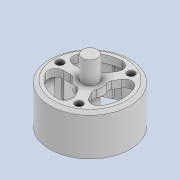
# Autodesk Inventor part: motor_1608_outer
Saved by Autodesk Inventor 2020 (Build 240168000, 168)
## iProperties
Created: 2020-01-30
Part Number: motor_1608_outer
Material: Generic
Document SubType Name: Modeling
Designer: psrobotics
Density: 1 g/cm^3
Appearance: Default
Author: psrobotics
Autodesk Inventor part; units mm, degrees
ref_plane "YZ Plane" through (0, 0, 0) normal (1, 0, 0) x (0, 1, 0)
ref_plane "XZ Plane" through (0, 0, 0) normal (0, 1, 0) x (-1, 0, 0)
ref_plane "XY Plane" through (0, 0, 0) normal (0, 0, 1) x (1, 0, 0)
sketch "Sketch1" plane through (0, 0, 0) normal (0, 1, 0) x (-1, 0, 0)
  circle A0 centre (0, 0) radius 8
  dimension "d0" = 16
  constraints: 1 centre point, 1 coincident
  measures "d0" diameter of A0
extrude "Extrusion1" add sketch "Sketch1" along normal blind 8
sketch "Sketch2" plane through (0, 8, 0) normal (0, 1, 0) x (1, 0, 0)
  circle A0 centre (0, 0) radius 8 projected
  circle A1 centre (0, 0) radius 1.5
  dimension "d3" = 3
  constraints: 1 centre point, 1 coincident
  measures "d3" diameter of A1
extrude "Extrusion2" add sketch "Sketch2" along normal blind 4.5 contours A1
sketch "Sketch3" plane through (0, 0, 0) normal (0, -1, 0) x (1, 0, 0)
  circle A0 centre (0, 0) radius 8 projected
  circle A1 centre (0, 0) radius 7.5
  dimension "d6" = 15
  constraints: 1 centre point, 1 coincident
  measures "d6" diameter of A1
extrude "Extrusion3" cut sketch "Sketch3" against normal blind 6.5 contours A1
sketch "Sketch4" plane through (0, 6.5, 0) normal (0, -1, 0) x (1, 0, 0)
  circle A0 centre (0, 0) radius 7.5 projected
  circle A1 centre (0, 0) radius 7
  line L0 (0, 0) -> (7.5, 0)
  circle A2 centre (0, 0) radius 7.5 projected
  line L1 (0, 0) -> (6.9038, -2.9305)
  point P0 (6.4435, -2.7351)
  point P1 (6.9038, -2.9305)
  point P2 (7, 0)
  dimension "d9" = 14
  dimension "d10" = 23
  constraints: 4 end point, 2 point on circle, 1 centre point, 1 coincident, 1 horizontal
  measures "d9" diameter of A1
  measures "d10" angle of L0 L1
extrude "Extrusion4" add sketch "Sketch4" along normal blind 6.2 contours A0 L1 A1 L0 picked at (6.8601, -2.5496)
pattern_circular "Circular Pattern1" count 10 over 360 about axis through (0, 0, 0) along (0, 1, 0) of "Extrusion4"
sketch "Sketch5" plane through (0, 8, 0) normal (0, 1, 0) x (1, 0, 0)
  circle A0 centre (0, 0) radius 2.5
  circle A1 centre (0, 0) radius 6.5
  line L0 (-10, -1) -> (-10, 1)
  line L1 (-10, 1) -> (10, 1)
  line L2 (10, 1) -> (10, -1)
  line L3 (10, -1) -> (-10, -1)
  line L4 (-10, -1) -> (10, 1) construction
  line L5 (-10, 1) -> (10, -1) construction
  line L6 (0, 0) -> (3.25, 5.6292)
  line L7 (0, 0) -> (-6.5, 0)
  line L8 (-5.866, -8.1603) -> (-4.134, -9.1603)
  line L9 (-4.134, -9.1603) -> (5.866, 8.1603)
  line L10 (5.866, 8.1603) -> (4.134, 9.1603)
  line L11 (4.134, 9.1603) -> (-5.866, -8.1603)
  line L12 (-5.866, -8.1603) -> (5.866, 8.1603) construction
  line L13 (-4.134, -9.1603) -> (4.134, 9.1603) construction
  point P0 (0.2796, 2.4843)
  point P1 (2.3453, 6.0621)
  point P2 (-6.4226, 1)
  point P3 (-2.2913, 1)
  dimension "d16" = 5
  dimension "d17" = 13
  dimension "d18" = 2
  dimension "d19" = 20
  dimension "d20" = 120
  dimension "d21" = 2
  dimension "d22" = 20
  constraints: 28 end point, 4 midpoint, 4 parallel, 3 perpendicular, 2 centre point, 2 coincident, 2 point on circle, 1 horizontal, 1 vertical
  measures "d16" diameter of A0
  measures "d17" diameter of A1
  measures "d18" distance of L0.start L0.end
  measures "d19" distance of L0.end L1.end
  measures "d20" angle of L7 L6
  measures "d21" distance of L8.start L8.end
  measures "d22" distance of L9.end L8.end
extrude "Extrusion5" cut sketch "Sketch5" against normal blind 6.2 contours A0 L1 A1 L11
pattern_circular "Circular Pattern2" count 3 over 360 about axis through (0, 8, 0) along (0, -1, 0) of "Extrusion5"
fillet "Fillet1" radius 1.5 2 edges at (-6.4226, 7.25, -1) (2.3453, 7.25, -6.0621)
pattern_circular "Circular Pattern3" count 3 over 360 about axis through (0, 8, 0) along (0, 1, 0) of "Fillet1"
fillet "Fillet2" radius 1 2 edges at (-2.2913, 7.25, -1) (0.2796, 7.25, -2.4843)
pattern_circular "Circular Pattern4" count 3 over 360 about axis through (0, 8, 0) along (0, 1, 0) of "Fillet2"
chamfer "Chamfer1" distance 0.8 angle 30 1 edges at (8, 8, 0) measured on face at (-6.1962, 8, 0)
sketch "Sketch6" plane through (0, 6.5, 0) normal (0, -1, 0) x (1, 0, 0)
  arc A0 (0, 6.5) -> (-5.6292, 3.25) centre (0, 0) ccw projected
  arc A1 (1.299, 4.25) -> (0, 6.5) centre (0, 5) ccw projected
  line L0 (1.299, 4.25) -> (0.5701, 2.9875) projected
  arc A2 (-0.2114, 2.491) -> (0.5701, 2.9875) centre (-0.2959, 3.4875) ccw projected
  arc A3 (-0.2114, 2.491) -> (-2.0516, 1.4286) centre (0, 0) ccw projected
  arc A4 (-2.8723, 1) -> (-2.0516, 1.4286) centre (-2.8723, 2) ccw projected
  line L1 (-2.8723, 1) -> (-4.3301, 1) projected
  arc A5 (-5.6292, 3.25) -> (-4.3301, 1) centre (-4.3301, 2.5) ccw projected
  arc A6 (5.6292, -3.25) -> (5.6292, 3.25) centre (0, 0) ccw projected
  arc A7 (3.0311, -3.25) -> (5.6292, -3.25) centre (4.3301, -2.5) ccw projected
  line L2 (3.0311, -3.25) -> (2.3022, -1.9875) projected
  arc A8 (2.263, -1.0625) -> (2.3022, -1.9875) centre (3.1682, -1.4875) ccw projected
  arc A9 (2.263, -1.0625) -> (2.263, 1.0625) centre (0, 0) ccw projected
  arc A10 (2.3022, 1.9875) -> (2.263, 1.0625) centre (3.1682, 1.4875) ccw projected
  line L3 (2.3022, 1.9875) -> (3.0311, 3.25) projected
  arc A11 (5.6292, 3.25) -> (3.0311, 3.25) centre (4.3301, 2.5) ccw projected
  arc A12 (-5.6292, -3.25) -> (0, -6.5) centre (0, 0) ccw projected
  arc A13 (-4.3301, -1) -> (-5.6292, -3.25) centre (-4.3301, -2.5) ccw projected
  line L4 (-4.3301, -1) -> (-2.8723, -1) projected
  arc A14 (-2.0516, -1.4286) -> (-2.8723, -1) centre (-2.8723, -2) ccw projected
  arc A15 (-2.0516, -1.4286) -> (-0.2114, -2.491) centre (0, 0) ccw projected
  arc A16 (0.5701, -2.9875) -> (-0.2114, -2.491) centre (-0.2959, -3.4875) ccw projected
  line L5 (0.5701, -2.9875) -> (1.299, -4.25) projected
  arc A17 (0, -6.5) -> (1.299, -4.25) centre (0, -5) ccw projected
  line L6 (7.3078, 1.6871) -> (6.8206, 1.5747) projected
  arc A18 (6.8206, 1.5747) -> (5.6631, 4.1145) centre (0, 0) ccw projected
  line L7 (5.6631, 4.1145) -> (6.0676, 4.4084) projected
  arc A19 (6.0676, 4.4084) -> (4.9204, 5.6603) centre (0, 0) ccw projected
  line L8 (4.9204, 5.6603) -> (4.5924, 5.283) projected
  arc A20 (4.5924, 5.283) -> (2.1631, 6.6574) centre (0, 0) ccw projected
  line L9 (2.1631, 6.6574) -> (2.3176, 7.1329) projected
  arc A21 (2.3176, 7.1329) -> (0.6537, 7.4715) centre (0, 0) ccw projected
  line L10 (0.6537, 7.4715) -> (0.6101, 6.9734) projected
  arc A22 (0.6101, 6.9734) -> (-2.1631, 6.6574) centre (0, 0) ccw projected
  line L11 (-2.1631, 6.6574) -> (-2.3176, 7.1329) projected
  arc A23 (-2.3176, 7.1329) -> (-3.8628, 6.4288) centre (0, 0) ccw projected
  line L12 (-3.8628, 6.4288) -> (-3.6053, 6.0002) projected
  arc A24 (-3.6053, 6.0002) -> (-5.6631, 4.1145) centre (0, 0) ccw projected
  line L13 (-5.6631, 4.1145) -> (-6.0676, 4.4084) projected
  arc A25 (-6.0676, 4.4084) -> (-6.9038, 2.9305) centre (0, 0) ccw projected
  line L14 (-6.9038, 2.9305) -> (-6.4435, 2.7351) projected
  arc A26 (-6.4435, 2.7351) -> (-7, 0) centre (0, 0) ccw projected
  line L15 (-7, 0) -> (-7.5, 0) projected
  arc A27 (-7.5, 0) -> (-7.3078, -1.6871) centre (0, 0) ccw projected
  line L16 (-7.3078, -1.6871) -> (-6.8206, -1.5747) projected
  arc A28 (-6.8206, -1.5747) -> (-5.6631, -4.1145) centre (0, 0) ccw projected
  line L17 (-5.6631, -4.1145) -> (-6.0676, -4.4084) projected
  arc A29 (-6.0676, -4.4084) -> (-4.9204, -5.6603) centre (0, 0) ccw projected
  line L18 (-4.9204, -5.6603) -> (-4.5924, -5.283) projected
  arc A30 (-4.5924, -5.283) -> (-2.1631, -6.6574) centre (0, 0) ccw projected
  line L19 (-2.1631, -6.6574) -> (-2.3176, -7.1329) projected
  arc A31 (-2.3176, -7.1329) -> (-0.6537, -7.4715) centre (0, 0) ccw projected
  line L20 (-0.6537, -7.4715) -> (-0.6101, -6.9734) projected
  arc A32 (-0.6101, -6.9734) -> (2.1631, -6.6574) centre (0, 0) ccw projected
  line L21 (2.1631, -6.6574) -> (2.3176, -7.1329) projected
  arc A33 (2.3176, -7.1329) -> (3.8628, -6.4288) centre (0, 0) ccw projected
  line L22 (3.8628, -6.4288) -> (3.6053, -6.0002) projected
  arc A34 (3.6053, -6.0002) -> (5.6631, -4.1145) centre (0, 0) ccw projected
  line L23 (5.6631, -4.1145) -> (6.0676, -4.4084) projected
  arc A35 (6.0676, -4.4084) -> (6.9038, -2.9305) centre (0, 0) ccw projected
  line L24 (6.9038, -2.9305) -> (6.4435, -2.7351) projected
  arc A36 (6.4435, -2.7351) -> (7, 0) centre (0, 0) ccw projected
  line L25 (7, 0) -> (7.5, 0) projected
  arc A37 (7.5, 0) -> (7.3078, 1.6871) centre (0, 0) ccw projected
  circle A38 centre (0, 0) radius 1.5
  dimension "d39" = 3
  constraints: 1 centre point, 1 coincident
  measures "d39" diameter of A38
extrude "Extrusion6" add sketch "Sketch6" along normal blind 5 contours A38
sketch "Sketch7" plane through (0, 8, 0) normal (0, 1, 0) x (1, 0, 0)
  circle A0 centre (0, 0) radius 1.5 projected
  arc A1 (0, 6.5) -> (-5.6292, 3.25) centre (0, 0) ccw projected
  arc A2 (1.299, 4.25) -> (0, 6.5) centre (0, 5) ccw projected
  line L0 (1.299, 4.25) -> (0.5701, 2.9875) projected
  arc A3 (-0.2114, 2.491) -> (0.5701, 2.9875) centre (-0.2959, 3.4875) ccw projected
  arc A4 (-0.2114, 2.491) -> (-2.0516, 1.4286) centre (0, 0) ccw projected
  arc A5 (-2.8723, 1) -> (-2.0516, 1.4286) centre (-2.8723, 2) ccw projected
  line L1 (-2.8723, 1) -> (-4.3301, 1) projected
  arc A6 (-5.6292, 3.25) -> (-4.3301, 1) centre (-4.3301, 2.5) ccw projected
  arc A7 (5.6292, -3.25) -> (5.6292, 3.25) centre (0, 0) ccw projected
  arc A8 (3.0311, -3.25) -> (5.6292, -3.25) centre (4.3301, -2.5) ccw projected
  line L2 (3.0311, -3.25) -> (2.3022, -1.9875) projected
  arc A9 (2.263, -1.0625) -> (2.3022, -1.9875) centre (3.1682, -1.4875) ccw projected
  arc A10 (2.263, -1.0625) -> (2.263, 1.0625) centre (0, 0) ccw projected
  arc A11 (2.3022, 1.9875) -> (2.263, 1.0625) centre (3.1682, 1.4875) ccw projected
  line L3 (2.3022, 1.9875) -> (3.0311, 3.25) projected
  arc A12 (5.6292, 3.25) -> (3.0311, 3.25) centre (4.3301, 2.5) ccw projected
  arc A13 (-5.6292, -3.25) -> (0, -6.5) centre (0, 0) ccw projected
  arc A14 (-4.3301, -1) -> (-5.6292, -3.25) centre (-4.3301, -2.5) ccw projected
  line L4 (-4.3301, -1) -> (-2.8723, -1) projected
  arc A15 (-2.0516, -1.4286) -> (-2.8723, -1) centre (-2.8723, -2) ccw projected
  arc A16 (-2.0516, -1.4286) -> (-0.2114, -2.491) centre (0, 0) ccw projected
  arc A17 (0.5701, -2.9875) -> (-0.2114, -2.491) centre (-0.2959, -3.4875) ccw projected
  line L5 (0.5701, -2.9875) -> (1.299, -4.25) projected
  arc A18 (0, -6.5) -> (1.299, -4.25) centre (0, -5) ccw projected
  circle A19 centre (0, 0) radius 7.2 projected
  line L6 (0, 0) -> (-6, 0)
  circle A20 centre (-6, 0) radius 0.75
  dimension "d42" = 6
  dimension "d43" = 1.5
  constraints: 2 end point, 1 centre point, 1 coincident, 1 horizontal
  measures "d42" distance of L6.start L6.end
  measures "d43" diameter of A20
extrude "Extrusion7" cut sketch "Sketch7" against normal blind 5 contours A20
pattern_circular "Circular Pattern5" count 3 over 360 about axis through (0, 8, 0) along (0, 1, 0) of "Extrusion7"
body "Solid1"
